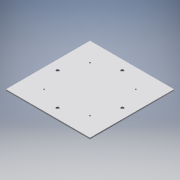
# Autodesk Inventor part: Top Plate
Saved by Autodesk Inventor 2016 (Build 200138000, 138)
## iProperties
Created: 2018-06-21
Part Number: Top Plate
Material: Generic
Document SubType Name: Modeling
Designer: Kade
Density: 1 g/cm^3
Appearance: Default
Mass: 130.479 g
Surface Area: 851.887 cm^2
Volume: 130.479 cm^3
Author: Kade
Autodesk Inventor part; units mm, degrees
ref_plane "YZ Plane" through (0, 0, 0) normal (1, 0, 0) x (0, 1, 0)
ref_plane "XZ Plane" through (0, 0, 0) normal (0, 1, 0) x (-1, 0, 0)
ref_plane "XY Plane" through (0, 0, 0) normal (0, 0, 1) x (1, 0, 0)
sketch "Sketch1" plane through (0, 0, 0) normal (0, 1, 0) x (-1, 0, 0)
  line L0 (-101.6, 101.6) -> (101.6, 101.6)
  line L1 (101.6, 101.6) -> (101.6, -101.6)
  line L2 (101.6, -101.6) -> (-101.6, -101.6)
  line L3 (-101.6, -101.6) -> (-101.6, 101.6)
  line L4 (-101.6, 101.6) -> (101.6, -101.6) construction
  line L5 (101.6, 101.6) -> (-101.6, -101.6) construction
  point P0 (0, 0)
  dimension "d0" = 203.2
  dimension "d1" = 203.2
  constraints: 12 end point, 2 midpoint, 2 parallel, 1 horizontal, 1 perpendicular
  measures "d0" distance of L1.end L2.end
  measures "d1" distance of L0.end L1.end
extrude "Extrusion1" add sketch "Sketch1" along normal blind 3.175
sketch "Sketch3" plane through (0, 3.175, 0) normal (0, 1, 0) x (1, 0, 0)
  circle A0 centre (0, -78.4352) radius 3.5719 projected
  circle A1 centre (78.4352, 0) radius 3.5719 projected
  circle A2 centre (0, 78.4352) radius 3.5719 projected
  circle A3 centre (-78.4352, 0) radius 3.5719 projected
  circle A4 centre (-55.4621, -55.4621) radius 1.651 projected
  circle A5 centre (55.4621, -55.4621) radius 1.651 projected
  circle A6 centre (55.4621, 55.4621) radius 1.651 projected
  circle A7 centre (-55.4621, 55.4621) radius 1.651 projected
  point P0 (0, 0)
extrude "Extrusion2" cut sketch "Sketch3" against normal through all
body "Solid1"
